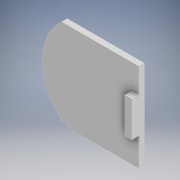
# Autodesk Inventor part: Case_Top_Slide
Saved by Autodesk Inventor 2020 (Build 240168000, 168)
## iProperties
Created: 2020-07-23
Part Number: Case_Top_Slide
Material: 일반
Document SubType Name: Modeling
Designer: Knowblesse
Density: 1 g/cm^3
Appearance: 기본값
Author: Knowblesse
## iProperties of the stored document _3D 인쇄.ipt
Created: 2020-07-23
Part Number: _3D 인쇄
Material: 일반
Document SubType Name: Modeling
Designer: Knowblesse
Density: 1 g/cm^3
Appearance: 기본값
Author: Knowblesse
Autodesk Inventor part; units mm, degrees
ref_plane "YZ Plane" through (0, 0, 0) normal (1, 0, 0) x (0, 1, 0)
ref_plane "XZ Plane" through (0, 0, 0) normal (0, 1, 0) x (-1, 0, 0)
ref_plane "XY Plane" through (0, 0, 0) normal (0, 0, 1) x (1, 0, 0)
sketch "스케치1" plane through (0, 0, 0) normal (0, 0, 1) x (1, 0, 0)
  line L0 (10.9058, 12.05) -> (0, 12.05)
  arc A0 (0, 12.05) -> (0, 0) centre (5.4138, 6.025) ccw
  line L1 (0, 0) -> (0.8, 0)
  line L2 (0.8, 0) -> (0.8, -0.45)
  line L3 (0.8, -0.45) -> (10.9058, -0.45)
  line L4 (10.9058, -0.45) -> (10.9058, 12.05)
  dimension "d0" = 8.1
  dimension "d1" = 12.5
  dimension "d2" = 5.492
  dimension "d3" = 0.45
  dimension "d4" = 0.8
  constraints: 10 end point, 3 perpendicular, 2 horizontal, 2 point on circle, 1 centre point, 1 vertical alignment
  measures "d0" radius of A0
  measures "d1" distance between parallel lines of L3 L0
  measures "d2" distance from line of A0.centre L4
  measures "d3" distance between parallel lines of L1 L3
  measures "d4" distance from line of L1.start L2
extrude "돌출1" add sketch "스케치1" along normal blind 0.8
sketch "스케치2" plane through (0, 0, 0.8) normal (0, 0, 1) x (1, 0, 0)
  line L0 (10.9058, -0.45) -> (10.9058, 12.05) projected
  arc A0 (0, 12.05) -> (0, 0) centre (5.4138, 6.025) ccw projected
  line L1 (9.9058, 8.525) -> (10.9058, 8.525)
  line L2 (10.9058, 8.525) -> (10.9058, 3.525)
  line L3 (10.9058, 3.525) -> (9.9058, 3.525)
  line L4 (9.9058, 3.525) -> (9.9058, 8.525)
  point P0 (9.9058, 6.025)
  dimension "d7" = 1
  dimension "d8" = 5
  constraints: 8 end point, 2 parallel, 1 collinear, 1 horizontal, 1 horizontal alignment, 1 midpoint, 1 perpendicular
  measures "d7" distance of L1.start L1.end
  measures "d8" distance between parallel lines of L1 L3
extrude "돌출2" add sketch "스케치2" along normal blind 1
